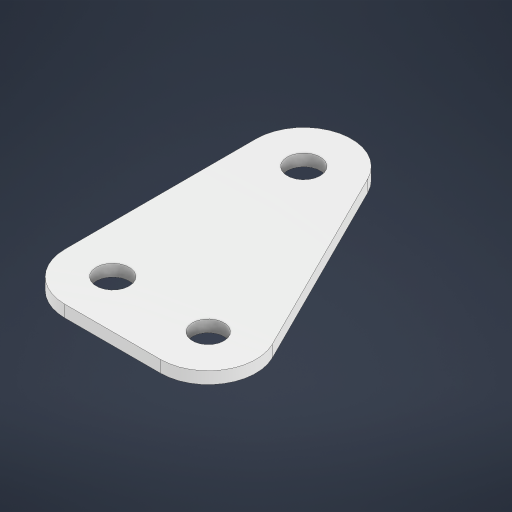
# Autodesk Inventor part: wing_pivot
Saved by Autodesk Inventor 2024 (Build 280153000, 153)
## iProperties
Created: 2023-10-18
Part Number: wing_pivot
Material: Acetal Resin, White
Document SubType Name: Sheet Metal
Designer: Averey Ku
Density: 1.425 g/cm^3
Flat Pattern Width: 2.40592 cm
Flat Pattern Length: 4.10981 cm
Flat Pattern Area: 9.88788 cm^2
Sheet Metal Rule: Default_mm
Sheet Metal Width: 0.947 in
Sheet Metal Length: 1.618 in
Sheet Metal Area: 1.533 in^2
Appearance: Smooth - White
Author: Averey Ku
Autodesk Inventor part; units mm, degrees
ref_plane "YZ Plane" through (0, 0, 0) normal (1, 0, 0) x (0, 1, 0)
ref_plane "XZ Plane" through (0, 0, 0) normal (0, 1, 0) x (-1, 0, 0)
ref_plane "XY Plane" through (0, 0, 0) normal (0, 0, 1) x (1, 0, 0)
sketch "Sketch1" plane through (0, 0, 0) normal (0, 1, 0) x (-1, 0, 0)
  circle A0 centre (0, 0) radius 2.1844
  circle A1 centre (0, -25.4) radius 2.1844
  arc A2 (6.35, 0) -> (0, 6.35) centre (0, 0) ccw
  arc A3 (-5.6796, -28.2398) -> (6.35, -25.4) centre (0, -25.4) ccw
  line L0 (6.35, 0) -> (6.35, -25.4)
  circle A4 centre (-12.7, 0) radius 2.0955
  arc A5 (-12.7, 6.35) -> (-18.3796, -2.8398) centre (-12.7, 0) ccw
  line L1 (0, 6.35) -> (-12.7, 6.35)
  line L2 (-18.3796, -2.8398) -> (-5.6796, -28.2398)
  dimension "d0" = 4.3688
  dimension "d1" = 12.7
  dimension "d2" = 4.191
  constraints: 6 centre point, 6 end point, 6 point on circle, 5 tangent, 4 coincident, 2 other
  measures "d0" diameter of A0
  measures "d1" diameter of A2
  measures "d2" diameter of A4
extrude "Extrusion1" add sketch "Sketch1" along normal blind 1.5875
equation "\"BendRadius\" = Thickness"
equation "\"BendReliefWidth\" = Thickness"
equation "\"BendReliefDepth\" = 0.5 * Thickness"
equation "\"CornerReliefSize\" = 4 * Thickness"
equation "\"MinimumRemnant\" = 2 * Thickness"
equation "\"TransitionRadius\" = BendRadius"
equation "\"JacobiRadiusSize\" = BendRadius"
equation "\"GapSize\" = Thickness"
equation "\"Thickness\" = 1.5875"
body "Solid1"
